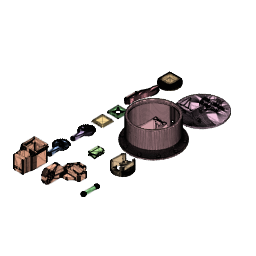
Pezzi+Singoli+Braccio+Robotico (Autodesk Fusion 360 design; units mm, degrees)
Autodesk Fusion 360 part; units mm, degrees
other "Base Mesh Feature1"
other "Base Mesh Feature2"
other "Base Mesh Feature3"
other "Base Mesh Feature4"
other "Base Mesh Feature5"
other "Base Mesh Feature6"
other "Base Mesh Feature7"
other "Base Mesh Feature8"
other "Base Mesh Feature9"
other "Base Mesh Feature10"
other "Base Mesh Feature11"
other "Base Mesh Feature12"
other "Base Mesh Feature13"
sketch "Sketch1" plane through (0, 0, 0) normal (0, 0, 1) x (1, 0, 0)
  line L0 (0, 0) -> (500, 0)
  line L1 (500, 0) -> (500, 500)
  line L2 (500, 500) -> (0, 500)
  line L3 (0, 500) -> (0, 0)
  dimension "d1" = 500
  dimension "d2" = 500
  constraint horizontal L0
  constraint vertical L1
  constraint horizontal L2
  constraint vertical L3
  constraint coincident L0.start L3.end
  measures "d1" distance of L0.start L0.end
  measures "d2" distance of L0.start L2.end
extrude "Extrude1" add sketch "Sketch1" against normal blind 25
other "Modify1"
other "Modify2"
other "Modify3"
other "Modify4"
other "Modify5"
other "Modify6"
other "Modify7"
other "Modify8"
other "Modify9"
other "Modify10"
other "Modify11"
other "Modify12"
other "Modify13"
other "Modify14"
other "Modify15"
other "Modify16"
other "Modify17"
other "Modify18"
move_body "Move1" bodies 1 to x (1, 0, 0) y (0, 1, 0) z (0, 0, 1) at (0, 0, -50)
other "Modify19"
other "Modify20"
other "Modify21"
other "Modify22"
other "Modify23"
other "Modify24"
other "Modify25"
other "Modify26"
other "Modify27"
other "Modify28"
other "Modify29"
other "Modify30"
other "Modify31"
other "Modify32"
other "Modify33"
other "Modify34"
other "Modify35"
other "Modify36"
other "Modify37"
other "Modify38"
other "Modify39"
other "Modify40"
other "Modify41"
other "Modify42"
other "Modify43"
other "Modify44"
other "Modify45"
other "Modify46"
other "Modify47"
other "Modify48"
other "Modify49"
hidden bodies 1
